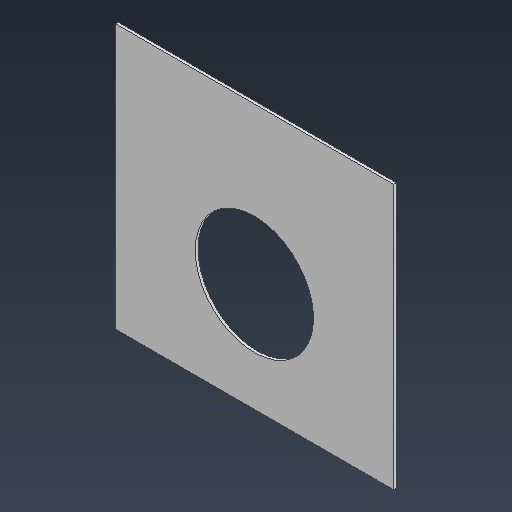
# Autodesk Inventor part: второй верх
Saved by Autodesk Inventor 2026 (Build 300175000, 175)
## iProperties
Created: 2025-11-21
Part Number: второй верх
Material: Типовые
Document SubType Name: Modeling
Designer: Phantom
Density: 1 g/cm^3
Appearance: По умолчанию
Author: Phantom
Autodesk Inventor part; units mm, degrees
ref_plane "YZ Plane" through (0, 0, 0) normal (1, 0, 0) x (0, 1, 0)
ref_plane "XZ Plane" through (0, 0, 0) normal (0, 1, 0) x (-1, 0, 0)
ref_plane "XY Plane" through (0, 0, 0) normal (0, 0, 1) x (1, 0, 0)
sketch "Эскиз1" plane through (0, 0, 0) normal (0, 0, 1) x (1, 0, 0)
  line L0 (-202.5, -190) -> (202.5, -190)
  line L1 (202.5, -190) -> (202.5, 190)
  line L2 (202.5, 190) -> (-202.5, 190)
  line L3 (-202.5, 190) -> (-202.5, -190)
  line L4 (-202.5, -190) -> (202.5, 190) construction
  line L5 (202.5, -190) -> (-202.5, 190) construction
  point P0 (0, 0)
  dimension "d0" = 405
  dimension "d1" = 380
  constraints: 12 end point, 2 midpoint, 2 parallel, 1 horizontal, 1 perpendicular
  measures "d0" distance of L2.end L1.end
  measures "d1" distance of L1.end L0.end
extrude "Выдавливание1" add sketch "Эскиз1" along normal blind 4
sketch "Эскиз2" plane through (0, 0, 4) normal (0, 0, 1) x (1, 0, 0)
  line L0 (-202.5, -190) -> (202.5, -190) projected
  line L1 (80, -190) -> (-80, -190)
  circle A0 centre (-0.87, -20.3549) radius 67.5 projected
  point P0 (0, 0)
  point P1 (0, -80)
  constraints: 2 end point, 1 point on line
extrude "Выдавливание2" cut sketch "Эскиз2" against normal blind 10
sketch "Эскиз3" plane through (0, 0, 0) normal (0, 0, -1) x (-1, 0, 0)
  circle A0 centre (0.87, -20.3549) radius 67.5 projected
  circle A1 centre (0.87, -20.3549) radius 80
  point P0 (0, 0)
  dimension "d8" = 160
  constraints: 1 centre point, 1 coincident
  measures "d8" diameter of A1
extrude "Выдавливание3" cut sketch "Эскиз3" against normal blind 10 contours A0 | A1
sketch "Эскиз4" plane through (0, 0, 0) normal (0, 0, -1) x (-1, 0, 0)
  circle A0 centre (-61.1233, -73.4234) radius 2.15 projected
  circle A1 centre (0.87, -20.3549) radius 80 projected
  circle A2 centre (0.87, -20.3549) radius 81.6053
  circle A3 centre (-61.1233, -73.4234) radius 4.5
  circle A4 centre (0.87, -20.3549) radius 86
  point P0 (0, 0)
  dimension "d11" = 9
  dimension "d13" = 172
  constraints: 3 coincident, 2 centre point, 3 other
  measures "d11" diameter of A3
  measures "d13" diameter of A4
extrude "Выдавливание4" cut sketch "Эскиз4" against normal blind 9 contours A0 A1 | A0 A1 A3 | A1 A0 A2 | A0 A2 A3 A1 | A1 A3 A2 A0 | A2 A0 | A0 A2 A3 A4 | A3 A2 A1 | A1 A3 | A3 A4 A2
sketch "Эскиз5" plane through (0, 0, 4) normal (0, 0, 1) x (1, 0, 0)
  line L0 (29.9071, 104.345) -> (29.9071, 34.345) projected
  line L1 (54.63, -143.2364) -> (54.63, -104.4746) projected
  circle A0 centre (-0.87, -20.3549) radius 86 projected
  circle A1 centre (-0.87, -20.3549) radius 150
  line L2 (-79.2827, -52.318) -> (-79.2827, 70.0459) projected
  circle A2 centre (-79.2827, 8.864) radius 61.1819
  circle A3 centre (-0.0936, -20) radius 3.5 projected
  circle A4 centre (-0.0936, -20) radius 150.042
  circle A5 centre (131.7561, -125.6612) radius 19.349
  circle A6 centre (-0.0936, -20) radius 101.8508
  line L3 (131.7561, -125.6612) -> (-0.0936, -20)
  line L4 (131.7561, -125.6612) -> (172.0961, -157.9887)
  line L5 (131.7561, -125.6612) -> (135.6578, -128.7879)
  point P0 (0, 0)
  dimension "d16" = 300
  dimension "d18" = 5
  constraints: 6 end point, 4 centre point, 4 coincident, 1 collinear, 1 midpoint, 1 point on line, 1 tangent, 1 vertical alignment, 2 other
  measures "d16" diameter of A1
  measures "d18" distance of L3.start L5.end
sketch "Эскиз6" plane through (0, 0, 4) normal (0, 0, 1) x (1, 0, 0)
  circle A0 centre (-0.87, -20.3549) radius 86 projected
  circle A1 centre (-0.87, -20.3549) radius 115
  circle A2 centre (-0.87, -20.3549) radius 86 projected
  line L0 (202.5, -190) -> (202.5, 190) projected
  line L1 (202.5, 190) -> (-202.5, 190) projected
  line L2 (-202.5, 190) -> (-202.5, -190) projected
  line L3 (-202.5, -190) -> (202.5, -190) projected
  point P0 (0, 0)
  dimension "d19" = 230
  constraints: 1 centre point, 1 coincident
  measures "d19" diameter of A1
sketch "Эскиз7" plane through (0, 0, 4) normal (0, 0, 1) x (1, 0, 0)
  arc A0 (9.4386, -46.6264) -> (-10.3633, -172.0731) centre (-0.4372, -109.3537) ccw
  circle A1 centre (-0.87, -20.3549) radius 3.5
  circle A2 centre (-0.87, -20.3549) radius 152.4999
  circle A3 centre (-0.4372, -109.3537) radius 63.5
  circle A4 centre (-0.4372, -109.3537) radius 86
  point P0 (0, 0)
  dimension "d22" = 172
  constraints: 5 centre point, 3 coincident, 2 point on circle, 1 concentric, 1 tangent, 6 other
  measures "d22" diameter of A4
extrude "Выдавливание6" cut sketch "Эскиз7" against normal blind 10 contours A3 A0 | A2 A4 A1 | A2 A4 | A4 A1 picked at (67.11, -105.4847) picked at (-0.9783, -23.5168)
sketch "Эскиз8" plane through (0, 0, 4) normal (0, 0, 1) x (1, 0, 0)
  arc A0 (-74.2445, -65.2122) -> (-30.3066, -190) centre (-0.4372, -109.3537) ccw projected
  arc A1 (72.9373, -64.4965) -> (-74.2445, -65.2122) centre (-0.87, -20.3549) ccw projected
  arc A2 (29.4322, -190) -> (72.9373, -64.4965) centre (-0.4372, -109.3537) ccw projected
  line L0 (29.4322, -190) -> (202.5, -190) projected
  line L1 (202.5, -190) -> (202.5, 190) projected
  line L2 (202.5, 190) -> (-202.5, 190) projected
  line L3 (-202.5, 190) -> (-202.5, -190) projected
  line L4 (-202.5, -190) -> (-30.3066, -190) projected
  line L5 (-202.5, -190) -> (202.5, -190)
  line L6 (202.5, -190) -> (202.5, -267)
  line L7 (202.5, -267) -> (-202.5, -267)
  line L8 (-202.5, -267) -> (-202.5, -190)
  circle A3 centre (-0.4372, -109.3537) radius 86
  point P0 (0, 0)
  point P1 (29.4322, -190)
  point P2 (-30.3066, -190)
  point P3 (-74.2445, -65.2122)
  constraints: 8 end point, 2 parallel, 1 centre point, 1 coincident, 1 concentric, 1 horizontal, 1 perpendicular
extrude "Выдавливание7" add sketch "Эскиз8" against normal up to surface (4 mm away) contours A1 A3 | A3 L0 L6 L7 L8 L4
sketch "Эскиз9" plane through (0, 0, 4) normal (0, 0, 1) x (1, 0, 0)
  arc A0 (116.0938, 103.8041) -> (94.7702, 121.9299) centre (105.15, 112.5352) ccw
  arc A1 (95.4845, 101.0568) -> (-96.801, 101.3917) centre (-0.87, -20.3549) ccw
  circle A2 centre (105.15, 112.5352) radius 5.5
  circle A3 centre (-0.5878, 141.6448) radius 2.25
  arc A4 (6.9903, 144.1437) -> (-8.1573, 144.1701) centre (-0.5961, 136.9179) ccw
  arc A5 (70.0743, 117.4562) -> (-71.3338, 117.7025) centre (-0.87, -20.3549) ccw
  circle A6 centre (168.4048, -36.1407) radius 5.5
  arc A7 (167.9768, -50.1342) -> (170.5666, -22.3086) centre (168.4048, -36.1407) ccw
  circle A8 centre (-0.87, -20.3549) radius 184.0093
  line L0 (149.2288, -195.3706) -> (149.2288, -224.0484)
  line L1 (202.5, 190) -> (-202.5, 190) projected
  line L2 (182.3446, -37.4382) -> (202.5, 190)
  line L3 (182.3446, -37.4382) -> (202.5, -37.4382)
  line L4 (202.5, -37.4382) -> (-270, -37.4382)
  line L5 (-202.5, 190) -> (-202.5, -267) projected
  line L6 (202.5, -267) -> (202.5, 190) projected
  line L7 (-202.5, -267) -> (202.5, -267) projected
  circle A9 centre (-0.87, -20.3549) radius 184.0093
  circle A10 centre (-0.87, -20.3549) radius 202.4448
  point P0 (0, 0)
  constraints: 11 point on circle, 10 centre point, 8 end point, 3 coincident, 1 horizontal, 1 point on line, 1 vertical, 32 other
sketch "Эскиз11" plane through (0, 0, 4) normal (0, 0, 1) x (1, 0, 0)
  line L0 (202.5, 190) -> (-202.5, 190) projected
  line L1 (-202.5, 190) -> (202.5, 190)
  line L2 (202.5, 190) -> (202.5, 118)
  line L3 (202.5, 118) -> (-202.5, 118)
  line L4 (-202.5, 118) -> (-202.5, 190)
  point P0 (0, 0)
  dimension "d33" = 405
  dimension "d34" = 72
  constraints: 8 end point, 2 parallel, 1 horizontal, 1 perpendicular
  measures "d33" distance of L2.end L3.end
  measures "d34" distance of L1.end L2.end
extrude "Выдавливание9" cut sketch "Эскиз11" against normal blind 10
equation "\"d14\" = d11"
